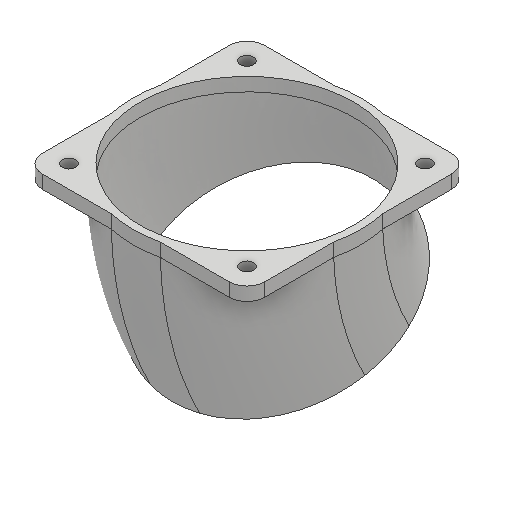
# Autodesk Inventor part: 3DP_ABS_Electronics_Colling_Tunnel
Saved by Autodesk Inventor 2026.1 (Build 301233000, 233)
## iProperties
Created: 2017-07-28
Part Number: 3DP_ABS_Electronics_Colling_Tunnel
Material: Ogólny
Document SubType Name: Modeling
Designer: Andrzej
Density: 1 g/cm^3
Appearance: Domyślna
Author: Andrzej
Autodesk Inventor part; units mm, degrees
ref_plane "YZ Plane" through (0, 0, 0) normal (1, 0, 0) x (0, 1, 0)
ref_plane "XZ Plane" through (0, 0, 0) normal (0, 1, 0) x (-1, 0, 0)
ref_plane "XY Plane" through (0, 0, 0) normal (0, 0, 1) x (1, 0, 0)
sketch "Szkic1" plane through (0, 0, 0) normal (0, 0, 1) x (1, 0, 0)
  circle A0 centre (0, 0) radius 24
  circle A1 centre (0, 0) radius 25.6
  line L0 (-21, 25) -> (-5.51, 25)
  line L1 (5.51, 25) -> (21, 25)
  line L2 (-25, -21) -> (-25, -5.51)
  line L3 (-25, 5.51) -> (-25, 21)
  line L4 (25, 21) -> (25, 5.51)
  line L5 (25, -5.51) -> (25, -21)
  line L6 (21, -25) -> (5.51, -25)
  line L7 (-5.51, -25) -> (-21, -25)
  arc A2 (-21, 25) -> (-25, 21) centre (-21, 21) ccw
  arc A3 (25, 21) -> (21, 25) centre (21, 21) ccw
  arc A4 (21, -25) -> (25, -21) centre (21, -21) ccw
  arc A5 (-25, -21) -> (-21, -25) centre (-21, -21) ccw
  point P0 (-25, 25)
  point P1 (25, -25)
  point P2 (25, 25)
  point P3 (-20, 20)
  point P4 (20, 20)
  point P5 (-20, -20)
  point P6 (20, -20)
  dimension "d0" = 48
  dimension "d1" = 50
  dimension "d2" = 50
  dimension "d5" = 40
  dimension "d6" = 40
  dimension "d7" = 20
  dimension "d8" = 20
  dimension "d9" = 1.6
  dimension "d10" = 4
  constraints: 16 end point, 8 parallel, 8 point on circle, 8 tangent, 6 point on line, 5 centre point, 4 perpendicular, 3 equal radius, 2 horizontal, 2 horizontal alignment, 2 vertical alignment, 1 coincident, 10 other
  measures "d0" diameter of A0
  measures "d1" distance of point (-25, 25) point (25, 25)
  measures "d2" distance of point (25, 25) point (25, -25)
  measures "d5" distance of point (20, 20) point (-20, 20)
  measures "d6" distance of point (-20, 20) point (-20, -20)
  measures "d7" horizontal distance of point (-20, 20) point (0, 0)
  measures "d8" horizontal distance of point (0, 0) point (-20, 20)
  measures "d10" radius of A2
sketch "Szkic2" plane through (0, 0, 0) normal (1, 0, 0) x (0, 1, 0)
  arc A0 (0, 0) -> (6.4705, -24.1481) centre (57.5642, 2.4833) ccw
  line L0 (0, 0) -> (6.4705, -24.1481) construction
  line L1 (0, 0) -> (25, 0) construction
  dimension "d11" = 25
  dimension "d12" = 75
  constraints: 4 end point, 2 point on circle, 1 centre point, 1 equal length, 1 horizontal
  measures "d11" distance of L0.start L0.end
  measures "d12" angle of L0 L1
sweep "Przeciągnięcie1" add profiles "Szkic1" path "Szkic2" contours A1
extrude "Wyciągnięcie proste1" add sketch "Szkic1" along normal blind 3
hole "Otwór1" at (-20, 20, 0) at (20, 20, 0) at (-20, -20, 0) at (20, -20, 0) direction (0, 0, 1) diameter 3 end through all
